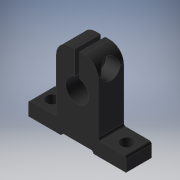
# Autodesk Inventor part: C-SHA10_b
Saved by Autodesk Inventor 2019 (Build 230136000, 136)
## iProperties
Created: 2022-11-15
Part Number: C-SHA10_b
Material: Generic
Catalog Web Link: www.cadenas.de
Description: C-SHA_base-Economy Shaft Supports - T-Shaped/Slit
Vendor: MISUMI
Document SubType Name: Modeling
Designer: psAdmin
Manufacturer: MISUMI
Mass: 6.44158 g
Surface Area: 37.5455 cm^2
Volume: 6.44158 cm^3
Density: 1 g/cm^3
Appearance: PSOLRGB-175-175-175
Category: PARTsolutions
Company: MISUMI
Title: C-SHA10
Author: Cadenas PARTsolutions
Comments: Economy Shaft Supports - T-Shaped/Slit
PSOL_IDENT_0: {$CADENAS_DATA/23d-libs/misumi/metric/02_shaft_supports/c_sha/c_sha_base.prj},160 {VTYP=3D},{NB=C-SH
PSOL_IDENT_1: A10_b},{LINA=C-SHA10},{NN=C-SHA_base},{DATE=04.10.2022 06:54:53},{GEOMDATE=23.04.2021 02:46:37},{VER
PSOL_IDENT_2: SION=},{LINEID=10},{WBVAR=},{WBNUMERIC=}  {NB=C-SHA10_b},{LINA=C-SHA10},{KT=DUMMY},{PN=C-SHA10},{TYP
PSOL_IDENT_3: E=C-SHA},{D=10},{H=20},{H1=35},{T=11},{L1=32},{DD=5.5},{E=9.5},{S=6},{R=6},{L=42},{B=14},{W=18},{M=M
PSOL_IDENT_4: 4},{R2=1},{W2=2.0},{M3D=4},{M3D2=6.0},{M3D3=8},{M3D4=4.3},{LB=10}
NB: C-SHA10_b
NN: C-SHA_base
NT: Economy Shaft Supports - T-Shaped/Slit
NBSYN: $PN._b
LINA: C-SHA10
CATALOG: Misumi
PN: C-SHA10
D: 10
H: 20
H1: 35
T: 11
L1: 32
DD: 5.5
E: 9.5
S: 6
R: 6
L: 42
B: 14
W: 18
M: M4
SUPPLIER: MISUMI
ARTICLENO: C-SHA10_b
BOMINFO: C-SHA10
CREATOR: CADENAS GmbH
Autodesk Inventor part; units mm, degrees
sketch "_____1" plane through (0, 0, 0) normal (0, 0, 1) x (1, 0, 0)
  line L0 (-21, -15) -> (-21, -20)
  line L1 (-21, -20) -> (-7, -20)
  arc A0 (-6, -19) -> (-7, -20) centre (-6, -20) ccw
  line L2 (-6, -19) -> (6, -19)
  arc A1 (7, -20) -> (6, -19) centre (6, -20) ccw
  line L3 (7, -20) -> (21, -20)
  line L4 (21, -20) -> (21, -15)
  arc A2 (21, -15) -> (20, -14) centre (20, -15) ccw
  line L5 (20, -14) -> (10, -14)
  arc A3 (9, -13) -> (10, -14) centre (10, -13) ccw
  line L6 (9, -13) -> (9, 9)
  arc A4 (9, 9) -> (3, 15) centre (3, 9) ccw
  line L7 (3, 15) -> (-3, 15)
  arc A5 (-3, 15) -> (-9, 9) centre (-3, 9) ccw
  line L8 (-9, 9) -> (-9, -13)
  arc A6 (-10, -14) -> (-9, -13) centre (-10, -13) ccw
  line L9 (-10, -14) -> (-20, -14)
  arc A7 (-20, -14) -> (-21, -15) centre (-20, -15) ccw
  constraints: 20 end point, 16 point on circle, 8 centre point
extrude "Extrusion1" add sketch "_____1" along normal mid plane 11
sketch "_____2" plane through (0, 0, 0) normal (0, 0, 1) x (1, 0, 0)
  arc A0 (-1, 4.899) -> (1, 4.899) centre (0, 0) ccw
  line L0 (1, 4.899) -> (1, 35)
  line L1 (1, 35) -> (-1, 35)
  line L2 (-1, 35) -> (-1, 4.899)
  constraints: 6 end point, 2 point on circle, 1 centre point
extrude "Extrusion2" cut sketch "_____2" along normal mid plane 11
sketch "_____3" plane through (0, 0, 0) normal (0, 1, 0) x (1, 0, 0)
  circle A0 centre (16, 0) radius 2.75
  constraints: 1 centre point
extrude "Extrusion3" cut sketch "_____3" against normal blind 20
sketch "_____4" plane through (0, 0, 0) normal (0, 1, 0) x (1, 0, 0)
  circle A0 centre (-16, 0) radius 2.75
  constraints: 1 centre point
extrude "Extrusion4" cut sketch "_____4" against normal blind 20
sketch "_____5" plane through (0, 0, 0) normal (0, 0, 1) x (1, 0, 0)
  line L0 (50, 9.5) -> (-50, 9.5)
  line L1 (0, 9.5) -> (0, 11.65)
  line L2 (0, 11.65) -> (3, 11.65)
  line L3 (3, 11.65) -> (3, 13.5)
  line L4 (3, 13.5) -> (9, 13.5)
  line L5 (9, 13.5) -> (9, 9.5)
  line L6 (9, 9.5) -> (0, 9.5)
  constraints: 14 end point
revolve "Revolution1" cut sketch "_____5" angle 360 about axis through (50, 9.5, 0) along (1, 0, 0)
sketch "Sketch6" plane through (-1, 4.899, 5.5) normal (1, 0, 0) x (0, 0, -1)
  point P0 (5.5, 4.601)
hole "Hole1" at (-1, 9.5, 0) direction (-1, 0, 0) diameter 3.242 depth 8 countersink diameter 4 countersink angle 90 thread size "M4x0.7" class "6H" standard "ISO Metric profile"
ref_plane "to_bolt_XY" through (3, 9.5, 0) normal (1, 0, 0) x (0, 0, -1)
ref_plane "to_bolt_YZ" through (3, 9.5, 0) normal (0, 0, -1) x (0, 1, 0)
ref_plane "to_bolt_ZX" through (3, 9.5, 0) normal (0, 1, 0) x (1, 0, 0)
body "Solid1"
